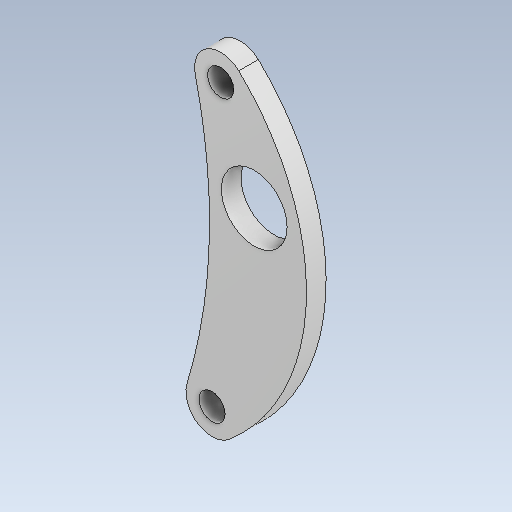
# Autodesk Inventor part: 原動節固定部
Saved by Autodesk Inventor 2020.4 (Build 244396000, 396)
## iProperties
Created: 2021-05-01
Part Number: 原動節固定部
Material: アルミニウム 2014-T4
Document SubType Name: Modeling
Designer: happy
Density: 2.8 g/cm^3
Appearance: サテン
Mass: 4.44387 g
Surface Area: 15.8362 cm^2
Volume: 1.5871 cm^3
Author: happy
Autodesk Inventor part; units mm, degrees
ref_plane "YZ Plane" through (0, 0, 0) normal (1, 0, 0) x (0, 1, 0)
ref_plane "XZ Plane" through (0, 0, 0) normal (0, 1, 0) x (-1, 0, 0)
ref_plane "XY Plane" through (0, 0, 0) normal (0, 0, 1) x (1, 0, 0)
sketch "スケッチ1" plane through (0, 0, 0) normal (0, 0, 1) x (1, 0, 0)
  circle A0 centre (154.8697, 39.0954) radius 2
  circle A1 centre (153.5524, -4.4926) radius 2
  circle A2 centre (160, 25) radius 2
  circle A3 centre (154.8697, 39.0954) radius 4
  circle A4 centre (153.5524, -4.4926) radius 4
  circle A5 centre (160, 25) radius 7
  circle A6 centre (160, 25) radius 5.025
  arc A7 (149.7263, -3.3259) -> (150.9802, 38.1619) centre (74.1465, 19.7211) ccw
  arc A8 (156.1251, -7.5554) -> (157.6227, 41.9973) centre (134.7514, 17.8895) ccw
  point P0 (0, 0)
  point P1 (0, 0)
  dimension "d0" = 8
  dimension "d1" = 8
  dimension "d2" = 14
  dimension "d3" = 10.05
  constraints: 9 centre point, 8 point on circle, 6 tangent, 4 coincident, 6 other
  measures "d0" diameter of A3
  measures "d1" diameter of A4
  measures "d2" diameter of A5
  measures "d3" diameter of A6
extrude "押し出し1" add sketch "スケッチ1" along normal blind 3 contours A3 | A3 A8 A5 A7 | A8 A4 A7 A5 | A5 | A4
